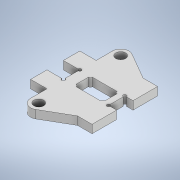
# Autodesk Inventor part: Part8
Saved by Autodesk Inventor 2021 (Build 250183000, 183)
## iProperties
Created: 2022-04-24
Part Number: Part8
Material: Generic
Document SubType Name: Modeling
Designer: hp
Density: 1 g/cm^3
Appearance: Default
Author: hp
Autodesk Inventor part; units mm, degrees
ref_plane "YZ Plane" through (0, 0, 0) normal (1, 0, 0) x (0, 1, 0)
ref_plane "XZ Plane" through (0, 0, 0) normal (0, 1, 0) x (-1, 0, 0)
ref_plane "XY Plane" through (0, 0, 0) normal (0, 0, 1) x (1, 0, 0)
sketch "Sketch1" plane through (0, 0, 0) normal (0, 1, 0) x (-1, 0, 0)
  line L0 (8, 10) -> (0, 10)
  line L1 (0, 10) -> (0, 40)
  line L2 (0, 40) -> (17.6795, 40)
  arc A0 (65, 50) -> (50, 58.6603) centre (55, 50) ccw
  line L3 (65, 50) -> (65, 40)
  line L4 (61.5, 0) -> (66, 0)
  line L5 (65, 40) -> (65, 30)
  line L6 (65, 30) -> (85, 30)
  line L7 (85, 30) -> (85, 0)
  line L8 (10, 8) -> (10, 0)
  line L9 (50, 58.6603) -> (17.6795, 40)
  circle A1 centre (55, 50) radius 6
  line L10 (85, 10) -> (65, 10)
  line L11 (65, 8) -> (65, 0)
  line L12 (85, 0) -> (85, 10)
  line L13 (52, 10) -> (17, 10)
  line L14 (17, 10) -> (17, 0)
  line L15 (17, 0) -> (52, 0)
  line L16 (52, 0) -> (52, 10)
  arc A2 (67, 10) -> (65, 8) centre (65, 10) ccw
  arc A3 (49.5, 10) -> (52, 7.5) centre (52, 10) ccw
  arc A4 (17, 7.5) -> (19.5, 10) centre (17, 10) ccw
  arc A5 (10, 8) -> (8, 10) centre (10, 10) ccw
  line L17 (8, -10) -> (0, -10)
  line L18 (0, -10) -> (0, -40)
  line L19 (0, -40) -> (17.6795, -40)
  arc A6 (50, -58.6603) -> (65, -50) centre (55, -50) ccw
  line L20 (65, -50) -> (65, -40)
  line L21 (65, -40) -> (65, -30)
  line L22 (65, -30) -> (85, -30)
  line L23 (85, -30) -> (85, 0)
  line L24 (10, -8) -> (10, 0)
  line L25 (50, -58.6603) -> (17.6795, -40)
  circle A7 centre (55, -50) radius 6
  line L26 (85, -10) -> (65, -10)
  line L27 (65, -8) -> (65, 0)
  line L28 (85, 0) -> (85, -10)
  line L29 (52, -10) -> (17, -10)
  line L30 (17, -10) -> (17, 0)
  line L31 (52, 0) -> (52, -10)
  arc A8 (65, -8) -> (67, -10) centre (65, -10) ccw
  arc A9 (52, -7.5) -> (49.5, -10) centre (52, -10) ccw
  arc A10 (19.5, -10) -> (17, -7.5) centre (17, -10) ccw
  arc A11 (8, -10) -> (10, -8) centre (10, -10) ccw
  point P0 (0, 0)
  dimension "d4" = 10
  dimension "d5" = 40
  dimension "d6" = 50
  dimension "d7" = 20
  dimension "d8" = 65
  dimension "d9" = 85
  dimension "d10" = 30
  dimension "d11" = 10
  dimension "d12" = 30
  dimension "d13" = 12
  dimension "d14" = 20
  dimension "d15" = 85
  dimension "d17" = 20
  dimension "d18" = 65
  dimension "d19" = 10
  dimension "d20" = 13
  dimension "d21" = 35
  dimension "d22" = 4
  dimension "d23" = 5
  dimension "d24" = 5
  dimension "d25" = 4
  constraints: 64 end point, 26 symmetric about line, 20 point on circle, 13 point on line, 12 centre point, 8 coincident, 5 perpendicular, 4 parallel, 3 horizontal, 2 tangent, 2 vertical, 6 other
  measures "d4" distance from line of point (0, 0) L0
  measures "d5" distance from line of point (0, 0) L2
  measures "d6" vertical distance of A0.centre point (0, 0)
  measures "d7" diameter of A0
  measures "d8" distance from line of point (0, 0) L3
  measures "d9" distance from line of point (0, 0) L7
  measures "d10" vertical distance of L6.end point (0, 0)
  measures "d11" horizontal distance of L8.start point (0, 0)
  measures "d12" angle of L9 L2
  measures "d13" diameter of A1
  measures "d14" distance between parallel lines of L5 L7
  measures "d15" distance between parallel lines of L1 L7
  measures "d17" distance of L10.start L10.end
  measures "d18" distance of point (0, 0) L11.end
  measures "d19" distance between parallel lines of L13 L15
  measures "d20" distance between parallel lines of L16 L11
  measures "d21" distance of L13.start L13.end
  measures "d22" diameter of A2
  measures "d23" diameter of A3
  measures "d24" diameter of A4
  measures "d25" diameter of A5
extrude "Extrusion1" add sketch "Sketch1" along normal blind 10 contours L0 L1 L2 L9 A0 L3 L5 L6 L7 L10 A2 L11 L27 A8 L26 L23 L22 L21 L20 A6 L25 L19 L18 L17 A11 L24 L8 A5 | L16 A3 L13 | A4 L14 L13 | L31 L29 A9 | A10 L29 L30
body "Solid1"
